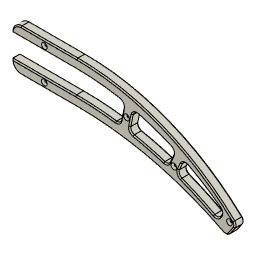
Tibia side mirrored (Autodesk Fusion 360 archive; units mm, degrees)
design "Tibia side"
Autodesk Fusion 360 part; units mm, degrees
note: some values were not read from the file. Set by a fixed rule: the direction of a hole.
sketch "Sketch1" plane through (0, 0, 0) normal (0, 1, 0) x (1, 0, 0)
  circle A0 centre (0, 0) radius 2.5
  line L0 (-10.1, -10) -> (29.9, -10)
  line L1 (29.9, -10) -> (29.9, 10)
  line L2 (29.9, 10) -> (-10.1, 10)
  line L3 (-10.1, 10) -> (-10.1, -10)
  line L4 (-10.1, -10) -> (-17.5, -10)
  line L5 (-17.5, -10) -> (-17.5, 10)
  line L6 (-17.5, 10) -> (-10.1, 10)
  line L7 (-10.1, 10) -> (-10.1, -10)
  line L8 (29.9, -10) -> (37.3, -10)
  line L9 (37.3, -10) -> (37.3, 10)
  line L10 (37.3, 10) -> (29.9, 10)
  line L11 (29.9, 10) -> (29.9, -10)
  line L12 (-18.6, -18.5) -> (38.4, -18.5)
  line L13 (38.4, -18.5) -> (38.4, 18.5) construction
  line L14 (38.4, 18.5) -> (-18.6, 18.5)
  line L15 (-18.6, 18.5) -> (-18.6, -18.5)
  line L16 (0, 0) -> (174.2843, 45) construction
  line L17 (169.9824, 51.1436) -> (178.5861, 38.8564)
  arc A1 (38.4, -18.5) -> (178.5861, 38.8564) centre (38.4, 181.4943) ccw
  arc A2 (38.4, 18.5) -> (169.9824, 51.1436) centre (38.4, 300.018) ccw
  line L18 (159.1401, 45.7067) -> (169.6952, 30.6325) construction
  arc A3 (37.3, -10) -> (167.1141, 34.3187) centre (37.3, 202.279) ccw
  arc A4 (37.3, 10) -> (161.7212, 42.0206) centre (37.3, 267.7398) ccw
  line L19 (161.7212, 42.0206) -> (167.1141, 34.3187)
  line L20 (76.2246, 12.9562) -> (80.0659, -5.6475)
  line L21 (84.1183, 14.2879) -> (87.8714, -3.8882)
  line L22 (118.3255, 23.0672) -> (124.5058, 8.7395)
  line L23 (125.8994, 25.7068) -> (131.7408, 12.165)
  line L24 (80.0659, -5.6475) -> (84.1183, 14.2879) construction
  line L25 (124.5058, 8.7395) -> (125.8994, 25.7068) construction
  line L26 (-17.5, -10) -> (-18.6, -10)
  line L27 (-17.5, 10) -> (-18.6, 10)
  line L28 (9.9, -10) -> (9.9, -18.5) construction
  line L29 (9.9, 10) -> (9.9, 18.5) construction
  line L30 (164.4176, 38.1696) -> (174.2843, 45) construction
  line L31 (162.5397, 53.0557) -> (179.3936, 28.9858) construction
  point P0 (174.2843, 45)
  point P1 (82.0921, 4.3202)
  point P2 (125.2026, 17.2232)
  point P3 (37.3, 0)
  point P4 (9.9, -13.85)
  point P5 (9.9, 13.85)
  point P6 (172.4675, 38.8774)
  point P7 (123.6183, 20.8961)
  dimension "d1" = 5
  dimension "d2" = 10.1
  dimension "d3" = 40
  dimension "d4" = 20
  dimension "d5" = 10
  dimension "d6" = 7.4
  dimension "d7" = 8.5
  dimension "d8" = 8.5
  dimension "d9" = 8.5
  dimension "d10" = 8.5
  dimension "d11" = 180
  dimension "d12" = 45
  dimension "d13" = 35
  dimension "d14" = 15
  dimension "d15" = 12
  dimension "d16" = 4.5
  dimension "d17" = 4.5
  dimension "d18" = 8
  dimension "d19" = 8
  dimension "d22" = 45
  dimension "d23" = 45
  dimension "d24" = 11.667
  dimension "d25" = 11.667
  dimension "d40" = 27.7
  dimension "d41" = 13.85
  dimension "d42" = 5
  dimension "d43" = 4
  dimension "d48" = 4
  dimension "d49" = 4
  constraint coincident A0.centre L16.start
  constraint horizontal L0
  constraint vertical L1
  constraint horizontal L2
  constraint vertical L3
  constraint horizontal L4
  constraint vertical L5
  constraint horizontal L6
  constraint vertical L7
  constraint horizontal L8
  constraint vertical L9
  constraint horizontal L10
  constraint vertical L11
  constraint coincident L2.end L3.start
  constraint coincident L1.end L2.start
  constraint equal L4 L8
  constraint horizontal L12
  constraint vertical L13
  constraint horizontal L14
  constraint vertical L15
  constraint coincident P0 L17
  constraint tangent L12 A1
  constraint tangent L14 A2
  constraint midpoint L17 P0
  constraint coincident P0 L16.end
  constraint parallel L17 L18
  constraint coincident L18 A3.end
  constraint tangent L8 A3
  constraint coincident L18 A4.end
  constraint tangent L10 A4
  constraint coincident A1 L18.end
  constraint coincident A2 L18.start
  constraint coincident A4 L20.start
  constraint coincident A3 L20.end
  constraint coincident A4 L21.start
  constraint coincident A3 L21.end
  constraint parallel L20 L21
  constraint coincident A4 L22.start
  constraint coincident A3 L22.end
  constraint coincident A4 L23.start
  constraint coincident A3 L23.end
  constraint parallel L22 L23
  constraint midpoint L24 P1
  constraint midpoint L25 P2
  constraint midpoint L9 P3
  constraint coincident L15 L26.end
  constraint perpendicular L15 L26
  constraint coincident L15 L27.end
  constraint perpendicular L15 L27
  constraint midpoint L0 L28.start
  constraint midpoint L12 L28.end
  constraint midpoint L2 L29.start
  constraint midpoint L14 L29.end
  constraint coincident L29 P5
  constraint midpoint L19 L30.start
  constraint parallel L17 L31
  constraint coincident L31 P6
  measures "d1" diameter of A0
  measures "d2" distance of A0.centre L3
  measures "d3" distance of L0.start L0.end
  measures "d4" distance of L0.end L1.end
  measures "d5" distance of A0.centre L0
  measures "d6" distance of L0.start L4.end
  measures "d7" distance of L7 L15
  measures "d8" distance of L1 L13
  measures "d9" distance of L2 L14
  measures "d10" distance of L0 L12
  measures "d11" distance of A0.centre P0
  measures "d12" vertical distance of A0.centre P0
  measures "d13" angle of L15 L17
  measures "d14" distance of L17.end L17.start
  measures "d15" distance of L17 L18
  measures "d16" distance of L18.end A3.end
  measures "d17" distance of L18.start A4.end
  measures "d18" distance of L20 L21
  measures "d19" distance of L22 L23
  measures "d22" distance of P1 P3
  measures "d23" distance of P1 P2
  measures "d24" angle of L9 L20
  measures "d25" angle of L21 L22
  measures "d40" distance of P4 P5
  measures "d41" vertical distance of A0.centre P5
  measures "d42" distance of L17 L31
  measures "d43" distance of L30 P6
  measures "d48" distance of P2 P7
  measures "d49" distance of L23 P7
extrude "Extrude1" add sketch "Sketch1" along normal blind 8 contours L0 L2 L4 L6 L8 L10 L12 L14 L15 L17 A1 A2 A3 A4 L19 L26 L27 | A3 A4 L20 L21 | A3 A4 L22 L23
hole "Hole1" at (82.0921, 0, -4.3202) at (9.9, 0, -13.85) at (9.9, 0, 13.85) at (172.4675, 0, -38.8774) at (123.6183, 0, -20.8961) direction (0, 1, 0) diameter 2 end through all countersink diameter 5 countersink angle 90
fillet "Fillet1" radius 4 2 edges at (178.5861, 4, -38.8564) (169.9824, 4, -51.1436)
fillet "Fillet2" radius 4 10 edges at (161.7212, 4, -42.0206) (167.1141, 4, -34.3187) (125.8994, 4, -25.7068) (131.7408, 4, -12.165) (118.3255, 4, -23.0672) (124.5058, 4, -8.7395) (84.1183, 4, -14.2879) (87.8714, 4, 3.8882) (80.0659, 4, 5.6475) (76.2246, 4, -12.9562)
fillet "Fillet3" radius 8 2 edges at (-18.6, 4, 18.5) (-18.6, 4, -18.5)
chamfer "Chamfer1" distance 1 angle 45 68 edges at (13.9, 0, 18.5) (112.5334, 0, 4.2527) (177.3303, 0, -38.9597) (174.3109, 0, -44.9619) (169.6806, 0, -49.8578) (104.4936, 0, -26.3686) (13.9, 0, -18.5) (-16.2569, 0, -16.1569) (-18.6, 0, -10.25) (-18.6, 0, 10.25) (-16.2569, 0, 16.1569) (13.9, 8, 18.5) (112.5334, 8, 4.2527) (177.3303, 8, -38.9597) (174.3109, 8, -44.9619) (169.6806, 8, -49.8578) (104.4936, 8, -26.3686) (13.9, 8, -18.5) (-16.2569, 8, -16.1569) (-18.6, 8, -10.25) (-18.6, 8, 10.25) (-16.2569, 8, 16.1569) (9.35, 0, -10) (9.35, 0, 10) (56.7628, 0, 9.1059) (78.6511, 0, 4.7297) (78.1177, 0, -3.7875) (75.3774, 0, -11.7227) (54.9529, 0, -10.6052) (101.5714, 0, -18.1421) (117.7573, 0, -21.7794) (121.3494, 0, -16.0569) (122.9745, 0, -9.3216) (106.5817, 0, -1.624) (88.8389, 0, 2.3771) (85.9808, 0, -5.268) (85.5192, 0, -13.3347) (144.4063, 0, -33.3085) (161.4224, 0, -40.6935) (164.3366, 0, -38.2853) (165.5776, 0, -34.541) (150.15, 0, -22.4812) (132.3866, 0, -13.8952) (128.8069, 0, -18.9664) (127.5479, 0, -24.988) (144.4063, 8, -33.3085) (161.4224, 8, -40.6935) (164.3366, 8, -38.2853) (165.5776, 8, -34.541) (150.15, 8, -22.4812) (132.3866, 8, -13.8952) (128.8069, 8, -18.9664) (127.5479, 8, -24.988) (101.5714, 8, -18.1421) (117.7573, 8, -21.7794) (121.3494, 8, -16.0569) (122.9745, 8, -9.3216) (106.5817, 8, -1.624) (88.8389, 8, 2.3771) (85.9808, 8, -5.268) (85.5192, 8, -13.3347) (54.9529, 8, -10.6052) (75.3774, 8, -11.7227) (78.1177, 8, -3.7875) (78.6511, 8, 4.7297) (56.7628, 8, 9.1059) (9.35, 8, 10) (9.35, 8, -10)
sketch "Sketch2" plane through (0, 8, 0) normal (0, 1, 0) x (-1, 0, 0)
  arc A0 (-129.4404, -28.1037) -> (-158.1379, -41.2149) centre (-37.3, -267.7398) ccw
  arc A1 (-164.587, -39.6712) -> (-158.1379, -41.2149) centre (-160.4912, -36.8033) ccw
  line L0 (-164.587, -39.6712) -> (-165.7245, -38.0466)
  arc A2 (-164.6134, -31.1673) -> (-165.7245, -38.0466) centre (-161.6288, -35.1787) ccw
  arc A3 (-136.0395, -13.2328) -> (-164.6134, -31.1673) centre (-37.3, -202.279) ccw
  arc A4 (-129.1336, -15.6843) -> (-136.0395, -13.2328) centre (-133.7247, -17.6647) ccw
  line L1 (-129.1336, -15.6843) -> (-126.6438, -21.4564)
  arc A5 (-129.4404, -28.1037) -> (-126.6438, -21.4564) centre (-131.2349, -23.4368) ccw
  circle A6 centre (-172.4675, -38.8774) radius 1
  circle A7 centre (-9.9, -13.85) radius 1
  circle A8 centre (-82.0921, -4.3202) radius 1
  circle A9 centre (-9.9, 13.85) radius 1
  line L2 (17.5821, -11) -> (-37.3, -11)
  arc A10 (-37.3, -11) -> (-72.3862, -13.4087) centre (-37.3, -267.7398) ccw
  arc A11 (-77.9662, -9.4667) -> (-72.3862, -13.4087) centre (-73.0695, -8.4557) ccw
  line L3 (-77.9662, -9.4667) -> (-80.228, 1.4873)
  arc A12 (-76.2443, 7.4143) -> (-80.228, 1.4873) centre (-75.3313, 2.4983) ccw
  arc A13 (-37.3, 11) -> (-76.2443, 7.4143) centre (-37.3, -202.279) ccw
  line L4 (-37.3, 11) -> (17.5821, 11)
  arc A14 (17.5821, 11) -> (10.6, 17.5) centre (10.6, 10.5) ccw
  line L5 (10.6, 17.5) -> (-38.4, 17.5)
  arc A15 (-38.4, 17.5) -> (-175.416, -37.1844) centre (-38.4, -181.4943) ccw
  arc A16 (-175.416, -37.1844) -> (-175.8078, -41.0807) centre (-173.3503, -39.36) ccw
  line L6 (-175.8078, -41.0807) -> (-171.1757, -47.696)
  arc A17 (-171.1757, -47.696) -> (-167.3489, -48.6446) centre (-168.7182, -45.9753) ccw
  arc A18 (-38.4, -17.5) -> (-167.3489, -48.6446) centre (-38.4, -300.018) ccw
  line L7 (-38.4, -17.5) -> (10.6, -17.5)
  arc A19 (10.6, -17.5) -> (17.5821, -11) centre (10.6, -10.5) ccw
  arc A20 (-87.8704, -16.0297) -> (-114.5887, -22.9097) centre (-37.3, -267.7398) ccw
  arc A21 (-120.685, -20.122) -> (-114.5887, -22.9097) centre (-116.0939, -18.1416) ccw
  line L8 (-120.685, -20.122) -> (-123.8503, -12.784)
  arc A22 (-121.2267, -6.207) -> (-123.8503, -12.784) centre (-119.2592, -10.8036) ccw
  arc A23 (-92.2288, 3.8053) -> (-121.2267, -6.207) centre (-37.3, -202.279) ccw
  arc A24 (-86.0444, -0.0149) -> (-92.2288, 3.8053) centre (-90.9411, -1.026) ccw
  line L9 (-86.0444, -0.0149) -> (-83.9586, -10.1166)
  arc A25 (-87.8704, -16.0297) -> (-83.9586, -10.1166) centre (-88.8553, -11.1277) ccw
  line L10 (-162.5397, -53.0557) -> (-179.3936, -28.9858)
  line L11 (-164.4176, -38.1696) -> (-174.2843, -45)
  circle A26 centre (-167.8788, -45.4307) radius 2.1
  circle A27 centre (-123.6183, -20.8961) radius 1
  dimension "d44" = 4.2
  dimension "d45" = 4
  constraint coincident L10 A26.centre
  measures "d44" diameter of A26
  measures "d45" distance of L11 A26.centre
extrude "Extrude2" cut sketch "Sketch2" against normal blind 3.5 contours L10 A26 | L10 A26
equation "d5 = d4 / 2"
equation "d8 = d7"
equation "d9 = d7"
equation "d10 = d7"
equation "d17 = d16"
equation "d19 = d18"
equation "d20 = d13 / 3"
equation "d23 = d22"
equation "d24 = d13 / 3"
equation "d25 = d24"
equation "d41 = d40 / 2"
equation "d49 = d19 / 2"
